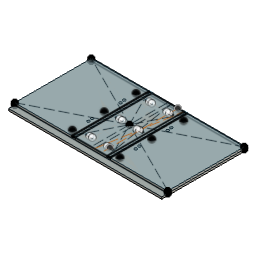
Table Saw Sled v13 (Autodesk Fusion 360 design; units mm, degrees)
Autodesk Fusion 360 part; units mm, degrees
sketch "Sketch1" plane through (0, 0, 0) normal (0, 0, 1) x (1, 0, 0)
  line L0 (0, 0) -> (914.4, 0)
  line L1 (914.4, 0) -> (914.4, 511.2)
  line L2 (914.4, 511.2) -> (0, 511.2)
  line L3 (0, 511.2) -> (0, 0)
  dimension "d1" = 914.4
  dimension "d2" = 511.2
  constraint horizontal L0
  constraint vertical L1
  constraint horizontal L2
  constraint vertical L3
  constraint coincident L0.start L3.end
  measures "d1" distance of L0.start L0.end
  measures "d2" distance of L0.start L2.end
extrude "Extrude1" add sketch "Sketch1" along normal blind 12 makes body 1
sketch "Sketch2" plane through (0, 0, 12) normal (0, 0, 1) x (-1, 0, 0)
  line L0 (0, -511.2) -> (0, 0)
  line L1 (0, 0) -> (-914.4, 0)
  line L2 (-914.4, 0) -> (-914.4, -511.2)
  line L3 (-914.4, -511.2) -> (0, -511.2)
  line L4 (0, 0) -> (-914.4, -511.2) construction
  line L5 (0, -511.2) -> (-914.4, 0) construction
  line L6 (-457.2, -511.2) -> (-457.2, 0) construction
  line L7 (-599.2812, -30.175) -> (-315.1187, -30.175) construction
  line L8 (-315.1187, -30.175) -> (-315.1187, -481.025) construction
  line L9 (-315.1187, -481.025) -> (-599.2812, -481.025) construction
  line L10 (-599.2812, -481.025) -> (-599.2812, -30.175) construction
  line L11 (-599.2812, -30.175) -> (-315.1187, -481.025) construction
  line L12 (-315.1187, -30.175) -> (-599.2812, -481.025) construction
  line L13 (-310.3562, -442.925) -> (-319.8812, -442.925)
  line L14 (-319.8812, -442.925) -> (-319.8812, -449.275)
  line L15 (-319.8812, -449.275) -> (-310.3562, -449.275)
  line L16 (-310.3562, -449.275) -> (-310.3562, -442.925)
  line L17 (-310.3562, -442.925) -> (-319.8812, -449.275) construction
  line L18 (-319.8812, -442.925) -> (-310.3562, -449.275) construction
  line L19 (-604.0438, -442.925) -> (-594.5188, -449.275) construction
  line L20 (-594.5188, -442.925) -> (-604.0438, -449.275) construction
  line L21 (-604.0438, -442.925) -> (-594.5188, -442.925)
  line L22 (-594.5188, -442.925) -> (-594.5188, -449.275)
  line L23 (-604.0438, -449.275) -> (-604.0438, -442.925)
  line L24 (-594.5188, -449.275) -> (-604.0438, -449.275)
  line L25 (-310.3562, -252.425) -> (-319.8812, -252.425)
  line L26 (-319.8812, -252.425) -> (-319.8812, -258.775)
  line L27 (-310.3562, -258.775) -> (-310.3562, -252.425)
  line L28 (-319.8812, -258.775) -> (-310.3562, -258.775)
  line L29 (-310.3562, -252.425) -> (-319.8812, -258.775) construction
  line L30 (-319.8812, -252.425) -> (-310.3562, -258.775) construction
  line L31 (-310.3562, -61.925) -> (-319.8812, -61.925)
  line L32 (-319.8812, -61.925) -> (-319.8812, -68.275)
  line L33 (-310.3562, -68.275) -> (-310.3562, -61.925)
  line L34 (-319.8812, -68.275) -> (-310.3562, -68.275)
  line L35 (-310.3562, -61.925) -> (-319.8812, -68.275) construction
  line L36 (-319.8812, -61.925) -> (-310.3562, -68.275) construction
  line L37 (-604.0438, -252.425) -> (-594.5188, -252.425)
  line L38 (-594.5188, -252.425) -> (-594.5188, -258.775)
  line L39 (-594.5188, -258.775) -> (-604.0438, -258.775)
  line L40 (-604.0438, -258.775) -> (-604.0438, -252.425)
  line L41 (-604.0438, -252.425) -> (-594.5188, -258.775) construction
  line L42 (-594.5188, -252.425) -> (-604.0438, -258.775) construction
  line L43 (-604.0438, -61.925) -> (-594.5188, -61.925)
  line L44 (-594.5188, -61.925) -> (-594.5188, -68.275)
  line L45 (-594.5188, -68.275) -> (-604.0438, -68.275)
  line L46 (-604.0438, -68.275) -> (-604.0438, -61.925)
  line L47 (-604.0438, -61.925) -> (-594.5188, -68.275) construction
  line L48 (-594.5188, -61.925) -> (-604.0438, -68.275) construction
  circle A0 centre (-316.7062, -350.85) radius 7.9375
  circle A1 centre (-316.7062, -160.35) radius 7.9375
  circle A2 centre (-313.5312, -185.75) radius 7.9375
  circle A3 centre (-313.5312, -376.25) radius 7.9375
  circle A4 centre (-597.6938, -374.25) radius 7.9375
  circle A5 centre (-600.8688, -348.85) radius 7.9375
  circle A6 centre (-597.6938, -183.75) radius 7.9375
  circle A7 centre (-600.8688, -158.35) radius 7.9375
  line L49 (-914.4, -255.6) -> (0, -255.6) construction
  line L50 (-31.75, -192.1) -> (-63.5, -192.1)
  line L51 (-63.5, -192.1) -> (-63.5, -319.1)
  line L52 (-63.5, -319.1) -> (-31.75, -319.1)
  line L53 (-31.75, -319.1) -> (-31.75, -192.1)
  line L54 (-31.75, -192.1) -> (-63.5, -319.1) construction
  line L55 (-63.5, -192.1) -> (-31.75, -319.1) construction
  line L56 (-882.65, -319.1) -> (-882.65, -192.1)
  line L57 (-882.65, -192.1) -> (-850.9, -192.1)
  line L58 (-850.9, -319.1) -> (-882.65, -319.1)
  line L59 (-850.9, -192.1) -> (-850.9, -319.1)
  line L60 (-850.9, -192.1) -> (-882.65, -319.1) construction
  line L61 (-882.65, -192.1) -> (-850.9, -319.1) construction
  point P0 (-457.2, -255.6)
  point P1 (-315.1187, -446.1)
  point P2 (-315.1187, -255.6)
  point P3 (-315.1187, -65.1)
  point P4 (-47.625, -255.6)
  point P5 (-866.775, -255.6)
  dimension "d5" = 284.1625
  dimension "d6" = 450.85
  dimension "d7" = 9.525
  dimension "d8" = 6.35
  dimension "d9" = 34.925
  dimension "d12" = 0
  dimension "d13" = 381
  dimension "d16" = 0
  dimension "d17" = 381
  dimension "d18" = 15.875
  dimension "d19" = 95.25
  dimension "d20" = 1.5875
  dimension "d21" = 15.875
  dimension "d22" = 95.25
  dimension "d23" = 1.5875
  dimension "d24" = 15.875
  dimension "d25" = 15.875
  dimension "d26" = 1.5875
  dimension "d27" = 1.5875
  dimension "d28" = 25.4
  dimension "d29" = 25.4
  dimension "d30" = 15.875
  dimension "d31" = 15.875
  dimension "d32" = 25.4
  dimension "d33" = 3.175
  dimension "d34" = 1.5875
  dimension "d35" = 15.875
  dimension "d36" = 15.875
  dimension "d37" = 25.4
  dimension "d38" = 3.175
  dimension "d39" = 1.5875
  dimension "d94" = 31.75
  dimension "d95" = 127
  dimension "d96" = 31.75
  constraint coincident L0.end L1.start
  constraint coincident L2.end L3.start
  constraint coincident L0.start L3.end
  constraint coincident L1.end L2.start
  constraint midpoint L3 L6.start
  constraint midpoint L1 L6.end
  constraint horizontal L7
  constraint perpendicular L7 L8
  constraint parallel L7 L9
  constraint parallel L8 L10
  constraint coincident L11 P0
  constraint coincident L12 P0
  constraint midpoint L5 P0
  constraint horizontal L13
  constraint perpendicular L13 L14
  constraint parallel L13 L15
  constraint parallel L14 L16
  constraint coincident L17 P1
  constraint coincident L18 P1
  constraint coincident L8 P1
  constraint symmetric L6 L13.start L19.start
  constraint symmetric L6 L13.end L20.start
  constraint symmetric L6 L14.end L19.end
  constraint symmetric L6 L15.end L20.end
  constraint midpoint L2 L49.start
  constraint midpoint L0 L49.end
  constraint horizontal L50
  constraint perpendicular L50 L51
  constraint parallel L50 L52
  constraint parallel L51 L53
  constraint coincident L54 P4
  constraint coincident L55 P4
  constraint coincident L49 P4
  constraint symmetric L6 L50.start L56.end
  constraint symmetric L6 L50.end L57.end
  constraint symmetric L6 L51.end L58.start
  constraint symmetric L6 L52.end L56.start
  constraint symmetric L6 P4 P5
  measures "d5" distance of L8.end L9.end
  measures "d6" distance of L7.end L8.end
  measures "d7" distance of L14.end L15.end
  measures "d8" distance of L13.end L14.end
  measures "d9" distance of L8.end P1
  measures "d18" diameter of A0
  measures "d19" vertical distance of P1 A0.centre
  measures "d20" distance of L8 A0.centre
  measures "d21" diameter of A1
  measures "d22" vertical distance of P3 A1.centre
  measures "d23" distance of L8 A1.centre
  measures "d24" diameter of A2
  measures "d25" diameter of A3
  measures "d26" distance of L8 A3.centre
  measures "d27" distance of L8 A2.centre
  measures "d28" vertical distance of A0.centre A3.centre
  measures "d29" vertical distance of A1.centre A2.centre
  measures "d30" diameter of A5
  measures "d31" diameter of A4
  measures "d32" vertical distance of A5.centre A4.centre
  measures "d33" horizontal distance of A5.centre A4.centre
  measures "d34" distance of L10 A4.centre
  measures "d35" diameter of A7
  measures "d36" diameter of A6
  measures "d37" vertical distance of A7.centre A6.centre
  measures "d38" horizontal distance of A7.centre A6.centre
  measures "d39" distance of L10 A6.centre
  measures "d94" distance of L51.end L52.end
  measures "d95" distance of L50.end L51.end
  measures "d96" distance of L0 L52.end
extrude "Extrude2" cut sketch "Sketch2" along normal through all and the other way through all contours L13 L14 L15 L16 | L21 L22 L23 L24 | L25 L26 L27 L28 | L31 L32 L33 L34 | L37 L38 L39 L40 | L43 L44 L45 L46 | A0 | A1 | A2 | A3 | A4 | A5 | A6 | A7 bodies 1
fillet "Fillet1" radius 3.175 24 edges at (310.3562, 449.275, 6) (310.3562, 258.775, 6) (594.5188, 258.775, 6) (594.5188, 449.275, 6) (310.3562, 68.275, 6) (594.5188, 68.275, 6) (319.8812, 61.925, 6) (604.0438, 61.925, 6) (604.0438, 252.425, 6) (604.0438, 442.925, 6) (319.8812, 442.925, 6) (319.8812, 252.425, 6) (604.0438, 258.775, 6) (319.8812, 258.775, 6) (319.8812, 68.275, 6) (319.8812, 449.275, 6) (604.0438, 449.275, 6) (604.0438, 68.275, 6) (310.3562, 252.425, 6) (310.3562, 442.925, 6) (594.5188, 442.925, 6) (594.5188, 252.425, 6) (594.5188, 61.925, 6) (310.3562, 61.925, 6) on bodies 1
copy_body "Body->Comp1" bodies 1 removing the originals makes body 2 in component "Component"
sketch "Sketch1 (2)" plane through (0, 0, 12) normal (0, 0, 1) x (-1, 0, 0) in component "Component'"
  circle A0 centre (-316.7062, -160.35) radius 7.9375
  arc A1 (-600.8688, -252.425) -> (-600.8688, -258.775) centre (-600.8688, -255.6) ccw
  line L0 (-600.8688, -252.425) -> (-597.6938, -252.425)
  arc A2 (-597.6938, -258.775) -> (-597.6938, -252.425) centre (-597.6938, -255.6) ccw
  line L1 (-597.6938, -258.775) -> (-600.8688, -258.775)
  line L2 (-313.5312, -449.275) -> (-316.7062, -449.275)
  arc A3 (-316.7062, -442.925) -> (-316.7062, -449.275) centre (-316.7062, -446.1) ccw
  line L3 (-316.7062, -442.925) -> (-313.5312, -442.925)
  arc A4 (-313.5312, -449.275) -> (-313.5312, -442.925) centre (-313.5312, -446.1) ccw
  circle A5 centre (-597.6938, -374.25) radius 7.9375
  circle A6 centre (-313.5312, -376.25) radius 7.9375
  circle A7 centre (-597.6938, -183.75) radius 7.9375
  arc A8 (-600.8688, -61.925) -> (-600.8688, -68.275) centre (-600.8688, -65.1) ccw
  line L4 (-600.8688, -61.925) -> (-597.6938, -61.925)
  arc A9 (-597.6938, -68.275) -> (-597.6938, -61.925) centre (-597.6938, -65.1) ccw
  line L5 (-597.6938, -68.275) -> (-600.8688, -68.275)
  circle A10 centre (-313.5312, -185.75) radius 7.9375
  arc A11 (-316.7062, -252.425) -> (-316.7062, -258.775) centre (-316.7062, -255.6) ccw
  line L6 (-316.7062, -252.425) -> (-313.5312, -252.425)
  arc A12 (-313.5312, -258.775) -> (-313.5312, -252.425) centre (-313.5312, -255.6) ccw
  line L7 (-313.5312, -258.775) -> (-316.7062, -258.775)
  line L8 (-597.6938, -449.275) -> (-600.8688, -449.275)
  arc A13 (-600.8688, -442.925) -> (-600.8688, -449.275) centre (-600.8688, -446.1) ccw
  line L9 (-600.8688, -442.925) -> (-597.6938, -442.925)
  arc A14 (-597.6938, -449.275) -> (-597.6938, -442.925) centre (-597.6938, -446.1) ccw
  circle A15 centre (-600.8688, -348.85) radius 7.9375
  circle A16 centre (-316.7062, -350.85) radius 7.9375
  circle A17 centre (-600.8688, -158.35) radius 7.9375
  arc A18 (-316.7062, -61.925) -> (-316.7062, -68.275) centre (-316.7062, -65.1) ccw
  line L10 (-316.7062, -61.925) -> (-313.5312, -61.925)
  arc A19 (-313.5312, -68.275) -> (-313.5312, -61.925) centre (-313.5312, -65.1) ccw
  line L11 (-313.5312, -68.275) -> (-316.7062, -68.275)
  line L12 (0, -511.2) -> (0, 0)
  line L13 (0, 0) -> (-914.4, 0)
  line L14 (-914.4, 0) -> (-914.4, -511.2)
  line L15 (-914.4, -511.2) -> (0, -511.2)
  line L16 (0, 0) -> (-914.4, 0)
  line L17 (-914.4, 0) -> (-914.4, -36)
  line L18 (-914.4, -36) -> (0, -36)
  line L19 (0, -36) -> (0, 0)
  dimension "d44" = 914.4
  dimension "d45" = 36
  constraint horizontal L16
  constraint vertical L17
  constraint horizontal L18
  constraint vertical L19
  constraint coincident L12.end L13.start
  measures "d44" distance of L12.end L13.end
  measures "d45" distance of L12.end L18.end
extrude "Extrude1'" add sketch "Sketch1 (2)" along normal blind 101.6 separate body contours L12 L13 L14 L16 L17 L18 L19 makes body 3 in component "Component'"
sketch "Sketch2 (2)" plane through (0, 0, 113.6) normal (0, 0, 1) x (-1, 0, 0) in component "Component'"
  line L0 (0, -36) -> (0, 0)
  line L1 (0, 0) -> (-914.4, 0)
  line L2 (-914.4, 0) -> (-914.4, -36)
  line L3 (-914.4, -36) -> (0, -36)
  line L4 (0, 0) -> (-914.4, -36) construction
  line L5 (-914.4, 0) -> (0, -36) construction
  line L6 (0, -18) -> (-914.4, -18)
  constraint coincident L0.end L1.start
  constraint coincident L2.end L3.start
  constraint coincident L1.end L2.start
  constraint coincident L0.start L3.end
  constraint midpoint L0 L6.start
  constraint midpoint L2 L6.end
extrude "Extrude2'" cut sketch "Sketch2 (2)" against normal blind 9.525 contours L0 L1 L2 L6 bodies 3 in component "Component'"
sketch "Sketch3" plane through (0, 0, 12) normal (0, 0, 1) x (-1, 0, 0) in component "Component'"
  circle A0 centre (-316.7062, -160.35) radius 7.9375
  arc A1 (-600.8688, -252.425) -> (-600.8688, -258.775) centre (-600.8688, -255.6) ccw
  line L0 (-600.8688, -252.425) -> (-597.6938, -252.425)
  arc A2 (-597.6938, -258.775) -> (-597.6938, -252.425) centre (-597.6938, -255.6) ccw
  line L1 (-597.6938, -258.775) -> (-600.8688, -258.775)
  line L2 (-313.5312, -449.275) -> (-316.7062, -449.275)
  arc A3 (-316.7062, -442.925) -> (-316.7062, -449.275) centre (-316.7062, -446.1) ccw
  line L3 (-316.7062, -442.925) -> (-313.5312, -442.925)
  arc A4 (-313.5312, -449.275) -> (-313.5312, -442.925) centre (-313.5312, -446.1) ccw
  circle A5 centre (-597.6938, -374.25) radius 7.9375
  circle A6 centre (-313.5312, -376.25) radius 7.9375
  circle A7 centre (-597.6938, -183.75) radius 7.9375
  arc A8 (-600.8688, -61.925) -> (-600.8688, -68.275) centre (-600.8688, -65.1) ccw
  line L4 (-600.8688, -61.925) -> (-597.6938, -61.925)
  arc A9 (-597.6938, -68.275) -> (-597.6938, -61.925) centre (-597.6938, -65.1) ccw
  line L5 (-597.6938, -68.275) -> (-600.8688, -68.275)
  circle A10 centre (-313.5312, -185.75) radius 7.9375
  arc A11 (-316.7062, -252.425) -> (-316.7062, -258.775) centre (-316.7062, -255.6) ccw
  line L6 (-316.7062, -252.425) -> (-313.5312, -252.425)
  arc A12 (-313.5312, -258.775) -> (-313.5312, -252.425) centre (-313.5312, -255.6) ccw
  line L7 (-313.5312, -258.775) -> (-316.7062, -258.775)
  line L8 (-597.6938, -449.275) -> (-600.8688, -449.275)
  arc A13 (-600.8688, -442.925) -> (-600.8688, -449.275) centre (-600.8688, -446.1) ccw
  line L9 (-600.8688, -442.925) -> (-597.6938, -442.925)
  arc A14 (-597.6938, -449.275) -> (-597.6938, -442.925) centre (-597.6938, -446.1) ccw
  circle A15 centre (-600.8688, -348.85) radius 7.9375
  circle A16 centre (-316.7062, -350.85) radius 7.9375
  circle A17 centre (-600.8688, -158.35) radius 7.9375
  arc A18 (-316.7062, -61.925) -> (-316.7062, -68.275) centre (-316.7062, -65.1) ccw
  line L10 (-316.7062, -61.925) -> (-313.5312, -61.925)
  arc A19 (-313.5312, -68.275) -> (-313.5312, -61.925) centre (-313.5312, -65.1) ccw
  line L11 (-313.5312, -68.275) -> (-316.7062, -68.275)
  line L12 (0, -511.2) -> (0, 0)
  line L13 (0, 0) -> (-914.4, 0)
  line L14 (-914.4, 0) -> (-914.4, -511.2)
  line L15 (-914.4, -511.2) -> (0, -511.2)
  line L16 (0, -511.2) -> (-914.4, -511.2)
  line L17 (-914.4, -511.2) -> (-914.4, -493.2)
  line L18 (-914.4, -493.2) -> (0, -493.2)
  line L19 (0, -493.2) -> (0, -511.2)
  dimension "d50" = 914.4
  dimension "d51" = 18
  constraint horizontal L16
  constraint vertical L17
  constraint horizontal L18
  constraint vertical L19
  constraint coincident L12.start L15.end
  measures "d50" distance of L12.start L14.end
  measures "d51" distance of L12.start L18.end
extrude "Extrude3" add sketch "Sketch3" along normal blind 101.6 separate body contours L12 L14 L15 L16 L17 L18 L19 makes body 4 in component "Component'"
sketch "Sketch4" plane through (0, 511.2, 0) normal (0, 1, 0) x (-1, 0, 0) in component "Component'"
  line L0 (-914.4, 12) -> (0, 12)
  line L1 (0, 12) -> (0, 113.6)
  line L2 (0, 113.6) -> (-914.4, 113.6)
  line L3 (-914.4, 113.6) -> (-914.4, 12)
  line L4 (-406.4, 12) -> (-508, 12)
  line L5 (-508, 12) -> (-508, 113.6)
  line L6 (-508, 113.6) -> (-406.4, 113.6)
  line L7 (-406.4, 113.6) -> (-406.4, 12)
  line L8 (-406.4, 12) -> (-508, 113.6) construction
  line L9 (-508, 12) -> (-406.4, 113.6) construction
  line L10 (-508, 113.6) -> (-558.8, 62.8)
  line L11 (-508, 113.6) -> (-436.158, 113.6) construction
  line L12 (-558.8, 62.8) -> (-914.4, 62.8)
  line L13 (-406.4, 113.6) -> (-355.6, 62.8)
  line L14 (-355.6, 62.8) -> (0, 62.8)
  point P0 (-457.2, 62.8)
  dimension "d54" = 101.6
  dimension "d55" = 135
  constraint horizontal L4
  constraint perpendicular L4 L5
  constraint parallel L4 L6
  constraint parallel L5 L7
  constraint coincident L8 P0
  constraint coincident L9 P0
  constraint horizontal L11
  constraint midpoint L3 L12.end
  constraint perpendicular L3 L12
  constraint perpendicular L9 L13
  constraint midpoint L1 L14.end
  constraint perpendicular L1 L14
  measures "d54" distance of L5.end L6.end
  measures "d55" angle of L10 L11
extrude "Extrude4" cut sketch "Sketch4" along normal through all and the other way up to surface (18 mm away) contours L2 L3 L10 L12 | L1 L2 L13 L14 bodies 4 in component "Component'"
sketch "Sketch2 (3)" plane through (0, 0, 12) normal (0, 0, 1) x (-1, 0, 0) in component "Component''"
  circle A0 centre (-316.7062, -160.35) radius 7.9375
  arc A1 (-600.8688, -252.425) -> (-600.8688, -258.775) centre (-600.8688, -255.6) ccw
  line L0 (-600.8688, -252.425) -> (-597.6938, -252.425)
  arc A2 (-597.6938, -258.775) -> (-597.6938, -252.425) centre (-597.6938, -255.6) ccw
  line L1 (-597.6938, -258.775) -> (-600.8688, -258.775)
  line L2 (-313.5312, -449.275) -> (-316.7062, -449.275)
  arc A3 (-316.7062, -442.925) -> (-316.7062, -449.275) centre (-316.7062, -446.1) ccw
  line L3 (-316.7062, -442.925) -> (-313.5312, -442.925)
  arc A4 (-313.5312, -449.275) -> (-313.5312, -442.925) centre (-313.5312, -446.1) ccw
  circle A5 centre (-597.6938, -374.25) radius 7.9375
  circle A6 centre (-313.5312, -376.25) radius 7.9375
  circle A7 centre (-597.6938, -183.75) radius 7.9375
  arc A8 (-600.8688, -61.925) -> (-600.8688, -68.275) centre (-600.8688, -65.1) ccw
  line L4 (-600.8688, -61.925) -> (-597.6938, -61.925)
  arc A9 (-597.6938, -68.275) -> (-597.6938, -61.925) centre (-597.6938, -65.1) ccw
  line L5 (-597.6938, -68.275) -> (-600.8688, -68.275)
  circle A10 centre (-313.5312, -185.75) radius 7.9375
  arc A11 (-316.7062, -252.425) -> (-316.7062, -258.775) centre (-316.7062, -255.6) ccw
  line L6 (-316.7062, -252.425) -> (-313.5312, -252.425)
  arc A12 (-313.5312, -258.775) -> (-313.5312, -252.425) centre (-313.5312, -255.6) ccw
  line L7 (-313.5312, -258.775) -> (-316.7062, -258.775)
  line L8 (-597.6938, -449.275) -> (-600.8688, -449.275)
  arc A13 (-600.8688, -442.925) -> (-600.8688, -449.275) centre (-600.8688, -446.1) ccw
  line L9 (-600.8688, -442.925) -> (-597.6938, -442.925)
  arc A14 (-597.6938, -449.275) -> (-597.6938, -442.925) centre (-597.6938, -446.1) ccw
  circle A15 centre (-600.8688, -348.85) radius 7.9375
  circle A16 centre (-316.7062, -350.85) radius 7.9375
  circle A17 centre (-600.8688, -158.35) radius 7.9375
  arc A18 (-316.7062, -61.925) -> (-316.7062, -68.275) centre (-316.7062, -65.1) ccw
  line L10 (-316.7062, -61.925) -> (-313.5312, -61.925)
  arc A19 (-313.5312, -68.275) -> (-313.5312, -61.925) centre (-313.5312, -65.1) ccw
  line L11 (-313.5312, -68.275) -> (-316.7062, -68.275)
  line L12 (0, -511.2) -> (0, 0)
  line L13 (0, 0) -> (-914.4, 0)
  line L14 (-914.4, 0) -> (-914.4, -511.2)
  line L15 (-914.4, -511.2) -> (0, -511.2)
  line L16 (0, -493.2) -> (-914.4, -493.2)
  line L17 (0, -36) -> (-914.4, -36)
  dimension "d60" = 36
  dimension "d61" = 18
  constraint coincident L12 L16.start
  constraint coincident L14 L16.end
  constraint perpendicular L14 L16
  constraint coincident L12 L17.start
  constraint coincident L14 L17.end
  constraint perpendicular L14 L17
  measures "d60" distance of L13 L17
  measures "d61" distance of L15 L16
extrude "Extrude1''" add sketch "Sketch2 (3)" along normal blind 12.7 separate body contours L12 L14 L16 L17 makes body 5 in component "Component''"
sketch "Sketch3 (2)" plane through (0, 0, 24.7) normal (0, 0, 1) x (-1, 0, 0) in component "Component''"
  circle A0 centre (-597.6938, -183.75) radius 7.9375
  arc A1 (-600.8688, -252.425) -> (-600.8688, -258.775) centre (-600.8688, -255.6) ccw
  line L0 (-600.8688, -252.425) -> (-597.6938, -252.425)
  arc A2 (-597.6938, -258.775) -> (-597.6938, -252.425) centre (-597.6938, -255.6) ccw
  line L1 (-597.6938, -258.775) -> (-600.8688, -258.775)
  arc A3 (-600.8688, -442.925) -> (-600.8688, -449.275) centre (-600.8688, -446.1) ccw
  line L2 (-600.8688, -442.925) -> (-597.6938, -442.925)
  arc A4 (-597.6938, -449.275) -> (-597.6938, -442.925) centre (-597.6938, -446.1) ccw
  line L3 (-597.6938, -449.275) -> (-600.8688, -449.275)
  circle A5 centre (-316.7062, -160.35) radius 7.9375
  circle A6 centre (-600.8688, -158.35) radius 7.9375
  arc A7 (-316.7062, -61.925) -> (-316.7062, -68.275) centre (-316.7062, -65.1) ccw
  line L4 (-316.7062, -61.925) -> (-313.5312, -61.925)
  arc A8 (-313.5312, -68.275) -> (-313.5312, -61.925) centre (-313.5312, -65.1) ccw
  line L5 (-313.5312, -68.275) -> (-316.7062, -68.275)
  arc A9 (-316.7062, -252.425) -> (-316.7062, -258.775) centre (-316.7062, -255.6) ccw
  line L6 (-316.7062, -252.425) -> (-313.5312, -252.425)
  arc A10 (-313.5312, -258.775) -> (-313.5312, -252.425) centre (-313.5312, -255.6) ccw
  line L7 (-313.5312, -258.775) -> (-316.7062, -258.775)
  circle A11 centre (-313.5312, -185.75) radius 7.9375
  arc A12 (-600.8688, -61.925) -> (-600.8688, -68.275) centre (-600.8688, -65.1) ccw
  line L8 (-600.8688, -61.925) -> (-597.6938, -61.925)
  arc A13 (-597.6938, -68.275) -> (-597.6938, -61.925) centre (-597.6938, -65.1) ccw
  line L9 (-597.6938, -68.275) -> (-600.8688, -68.275)
  circle A14 centre (-313.5312, -376.25) radius 7.9375
  circle A15 centre (-316.7062, -350.85) radius 7.9375
  arc A16 (-316.7062, -442.925) -> (-316.7062, -449.275) centre (-316.7062, -446.1) ccw
  line L10 (-316.7062, -442.925) -> (-313.5312, -442.925)
  arc A17 (-313.5312, -449.275) -> (-313.5312, -442.925) centre (-313.5312, -446.1) ccw
  line L11 (-313.5312, -449.275) -> (-316.7062, -449.275)
  circle A18 centre (-600.8688, -348.85) radius 7.9375
  circle A19 centre (-597.6938, -374.25) radius 7.9375
  line L12 (0, -493.2) -> (0, -36)
  line L13 (0, -36) -> (-914.4, -36)
  line L14 (-914.4, -36) -> (-914.4, -493.2)
  line L15 (-914.4, -493.2) -> (0, -493.2)
  arc A20 (-597.6938, -452.45) -> (-597.6938, -439.75) centre (-597.6938, -446.1) ccw
  line L16 (-600.8688, -439.75) -> (-597.6938, -439.75)
  arc A21 (-600.8688, -439.75) -> (-600.8688, -452.45) centre (-600.8688, -446.1) ccw
  line L17 (-597.6938, -452.45) -> (-600.8688, -452.45)
  arc A22 (-313.5312, -261.95) -> (-313.5312, -249.25) centre (-313.5312, -255.6) ccw
  line L18 (-316.7062, -249.25) -> (-313.5312, -249.25)
  arc A23 (-316.7062, -249.25) -> (-316.7062, -261.95) centre (-316.7062, -255.6) ccw
  line L19 (-313.5312, -261.95) -> (-316.7062, -261.95)
  arc A24 (-597.6938, -71.45) -> (-597.6938, -58.75) centre (-597.6938, -65.1) ccw
  line L20 (-600.8688, -58.75) -> (-597.6938, -58.75)
  arc A25 (-600.8688, -58.75) -> (-600.8688, -71.45) centre (-600.8688, -65.1) ccw
  line L21 (-597.6938, -71.45) -> (-600.8688, -71.45)
  arc A26 (-313.5312, -71.45) -> (-313.5312, -58.75) centre (-313.5312, -65.1) ccw
  line L22 (-316.7062, -58.75) -> (-313.5312, -58.75)
  arc A27 (-316.7062, -58.75) -> (-316.7062, -71.45) centre (-316.7062, -65.1) ccw
  line L23 (-313.5312, -71.45) -> (-316.7062, -71.45)
  arc A28 (-313.5312, -452.45) -> (-313.5312, -439.75) centre (-313.5312, -446.1) ccw
  line L24 (-316.7062, -439.75) -> (-313.5312, -439.75)
  arc A29 (-316.7062, -439.75) -> (-316.7062, -452.45) centre (-316.7062, -446.1) ccw
  line L25 (-313.5312, -452.45) -> (-316.7062, -452.45)
  arc A30 (-597.6938, -261.95) -> (-597.6938, -249.25) centre (-597.6938, -255.6) ccw
  line L26 (-600.8688, -249.25) -> (-597.6938, -249.25)
  arc A31 (-600.8688, -249.25) -> (-600.8688, -261.95) centre (-600.8688, -255.6) ccw
  line L27 (-597.6938, -261.95) -> (-600.8688, -261.95)
  dimension "d64" = -3.175
  measures "d64" distance of A4
extrude "Extrude2''" cut sketch "Sketch3 (2)" along normal blind -4.7625 and the other way blind 0 contours A20 L16 A21 L17 | A22 L18 A23 L19 | A24 L20 A25 L21 | A26 L22 A27 L23 | A28 L24 A29 L25 | A30 L26 A31 L27 bodies 5 in component "Component''"
sketch "Sketch4 (2)" plane through (0, 0, 24.7) normal (0, 0, 1) x (-1, 0, 0) in component "Component''"
  line L0 (-597.6938, -452.45) -> (-600.8688, -452.45)
  arc A0 (-600.8688, -439.75) -> (-600.8688, -452.45) centre (-600.8688, -446.1) ccw
  line L1 (-600.8688, -439.75) -> (-597.6938, -439.75)
  arc A1 (-597.6938, -452.45) -> (-597.6938, -439.75) centre (-597.6938, -446.1) ccw
  line L2 (-313.5312, -71.45) -> (-316.7062, -71.45)
  arc A2 (-316.7062, -58.75) -> (-316.7062, -71.45) centre (-316.7062, -65.1) ccw
  line L3 (-316.7062, -58.75) -> (-313.5312, -58.75)
  arc A3 (-313.5312, -71.45) -> (-313.5312, -58.75) centre (-313.5312, -65.1) ccw
  line L4 (-313.5312, -452.45) -> (-316.7062, -452.45)
  arc A4 (-316.7062, -439.75) -> (-316.7062, -452.45) centre (-316.7062, -446.1) ccw
  line L5 (-316.7062, -439.75) -> (-313.5312, -439.75)
  arc A5 (-313.5312, -452.45) -> (-313.5312, -439.75) centre (-313.5312, -446.1) ccw
  line L6 (-597.6938, -261.95) -> (-600.8688, -261.95)
  arc A6 (-600.8688, -249.25) -> (-600.8688, -261.95) centre (-600.8688, -255.6) ccw
  line L7 (-600.8688, -249.25) -> (-597.6938, -249.25)
  arc A7 (-597.6938, -261.95) -> (-597.6938, -249.25) centre (-597.6938, -255.6) ccw
  line L8 (-597.6938, -71.45) -> (-600.8688, -71.45)
  arc A8 (-600.8688, -58.75) -> (-600.8687, -71.45) centre (-600.8688, -65.1) ccw
  line L9 (-600.8688, -58.75) -> (-597.6938, -58.75)
  arc A9 (-597.6938, -71.45) -> (-597.6938, -58.75) centre (-597.6938, -65.1) ccw
  line L10 (-313.5312, -261.95) -> (-316.7062, -261.95)
  arc A10 (-316.7062, -249.25) -> (-316.7062, -261.95) centre (-316.7062, -255.6) ccw
  line L11 (-316.7062, -249.25) -> (-313.5312, -249.25)
  arc A11 (-313.5312, -261.95) -> (-313.5312, -249.25) centre (-313.5312, -255.6) ccw
  circle A12 centre (-597.6938, -183.75) radius 7.9375
  circle A13 centre (-316.7062, -160.35) radius 7.9375
  circle A14 centre (-600.8688, -158.35) radius 7.9375
  circle A15 centre (-313.5312, -185.75) radius 7.9375
  circle A16 centre (-313.5312, -376.25) radius 7.9375
  circle A17 centre (-316.7062, -350.85) radius 7.9375
  circle A18 centre (-600.8688, -348.85) radius 7.9375
  circle A19 centre (-597.6938, -374.25) radius 7.9375
  line L12 (0, -493.2) -> (0, -36)
  line L13 (0, -36) -> (-914.4, -36)
  line L14 (-914.4, -36) -> (-914.4, -493.2)
  line L15 (-914.4, -493.2) -> (0, -493.2)
  line L16 (0, -36) -> (-914.4, -493.2) construction
  line L17 (-914.4, -36) -> (0, -493.2) construction
  line L18 (-342.9, -493.2) -> (-571.5, -493.2)
  line L19 (-571.5, -493.2) -> (-571.5, -36)
  line L20 (-571.5, -36) -> (-342.9, -36)
  line L21 (-342.9, -36) -> (-342.9, -493.2)
  line L22 (-342.9, -493.2) -> (-571.5, -36) construction
  line L23 (-571.5, -493.2) -> (-342.9, -36) construction
  line L24 (-571.5, -36) -> (-552.45, -36)
  line L25 (-552.45, -36) -> (-552.45, -494.848)
  line L26 (-552.45, -494.848) -> (-571.5, -494.848)
  line L27 (-571.5, -494.848) -> (-571.5, -36)
  line L28 (-342.9, -36) -> (-361.95, -36)
  line L29 (-361.95, -36) -> (-361.95, -495.1951)
  line L30 (-361.95, -495.1951) -> (-342.9, -495.1951)
  line L31 (-342.9, -495.1951) -> (-342.9, -36)
  line L32 (-457.2, -493.2) -> (-457.2, -36) construction
  line L33 (-476.25, -493.2) -> (-476.25, -36) construction
  line L34 (-476.25, -36) -> (-552.45, -494.848) construction
  line L35 (-476.25, -493.2) -> (-552.45, -36) construction
  line L36 (-517.5749, -493.2) -> (-517.5749, -36) construction
  line L37 (-498.5249, -83.625) -> (-536.6249, -83.625)
  line L38 (-536.6249, -83.625) -> (-536.6249, -89.975)
  line L39 (-536.6249, -89.975) -> (-498.5249, -89.975)
  line L40 (-498.5249, -89.975) -> (-498.5249, -83.625)
  line L41 (-498.5249, -83.625) -> (-536.6249, -89.975) construction
  line L42 (-536.6249, -83.625) -> (-498.5249, -89.975) construction
  line L43 (-377.7751, -89.975) -> (-415.8751, -89.975)
  line L44 (-415.8751, -83.625) -> (-377.7751, -89.975) construction
  line L45 (-377.7751, -83.625) -> (-415.8751, -89.975) construction
  line L46 (-377.7751, -83.625) -> (-377.7751, -89.975)
  line L47 (-415.8751, -83.625) -> (-377.7751, -83.625)
  line L48 (-415.8751, -89.975) -> (-415.8751, -83.625)
  line L49 (-415.8751, -261.425) -> (-377.7751, -261.425)
  line L50 (-377.7751, -261.425) -> (-377.7751, -267.775)
  line L51 (-377.7751, -267.775) -> (-415.8751, -267.775)
  line L52 (-415.8751, -267.775) -> (-415.8751, -261.425)
  line L53 (-415.8751, -261.425) -> (-377.7751, -267.775) construction
  line L54 (-377.7751, -261.425) -> (-415.8751, -267.775) construction
  line L55 (-536.6249, -267.775) -> (-498.5249, -267.775)
  line L56 (-498.5249, -261.425) -> (-536.6249, -267.775) construction
  line L57 (-536.6249, -261.425) -> (-498.5249, -267.775) construction
  line L58 (-415.8751, -439.225) -> (-377.7751, -439.225)
  line L59 (-377.7751, -439.225) -> (-377.7751, -445.575)
  line L60 (-377.7751, -445.575) -> (-415.8751, -445.575)
  line L61 (-415.8751, -445.575) -> (-415.8751, -439.225)
  line L62 (-415.8751, -439.225) -> (-377.7751, -445.575) construction
  line L63 (-377.7751, -439.225) -> (-415.8751, -445.575) construction
  line L64 (-536.6249, -445.575) -> (-498.5249, -445.575)
  line L65 (-498.5249, -439.225) -> (-536.6249, -445.575) construction
  line L66 (-536.6249, -439.225) -> (-498.5249, -445.575) construction
  line L67 (-498.5249, -261.425) -> (-536.6249, -261.425)
  line L68 (-498.5249, -267.775) -> (-498.5249, -261.425)
  line L69 (-536.6249, -261.425) -> (-536.6249, -267.775)
  line L70 (-498.5249, -439.225) -> (-536.6249, -439.225)
  line L71 (-498.5249, -445.575) -> (-498.5249, -439.225)
  line L72 (-536.6249, -439.225) -> (-536.6249, -445.575)
  point P0 (-457.2, -264.6)
  point P1 (-517.5749, -86.8)
  point P2 (-396.8251, -86.8)
  point P3 (-396.8251, -264.6)
  point P4 (-517.5749, -264.6)
  point P5 (-396.8251, -442.4)
  point P6 (-517.5749, -442.4)
  point P7 (-412.7001, -86.8)
  point P8 (-412.7001, -264.6)
  point P9 (-412.7001, -442.4)
  point P10 (-501.6999, -86.8)
  point P11 (-501.6999, -264.6)
  point P12 (-501.6999, -442.4)
  dimension "d69" = 228.6
  dimension "d70" = 457.2
  dimension "d71" = 19.05
  dimension "d72" = 19.05
  dimension "d76" = 19.05
  dimension "d77" = 38.1
  dimension "d78" = 6.35
  dimension "d79" = 50.8
  dimension "d82" = 0
  dimension "d83" = -355.6
  dimension "d107" = 3.175
  constraint coincident L12.end L13.start
  constraint coincident L14.end L15.start
  constraint coincident L13.end L14.start
  constraint coincident L12.start L15.end
  constraint horizontal L18
  constraint perpendicular L18 L19
  constraint parallel L18 L20
  constraint parallel L19 L21
  constraint coincident L22 P0
  constraint coincident L23 P0
  constraint midpoint L16 P0
  constraint horizontal L24
  constraint vertical L25
  constraint horizontal L26
  constraint vertical L27
  constraint horizontal L28
  constraint vertical L29
  constraint horizontal L30
  constraint vertical L31
  constraint midpoint L18 L32.start
  constraint midpoint L20 L32.end
  constraint coincident L18 L33.start
  constraint coincident L20 L33.end
  constraint perpendicular L20 L33
  constraint coincident L15 L36.start
  constraint perpendicular L15 L36
  constraint coincident L20 L36.end
  constraint horizontal L37
  constraint perpendicular L37 L38
  constraint parallel L37 L39
  constraint parallel L38 L40
  constraint coincident L41 P1
  constraint coincident L42 P1
  constraint coincident L36 P1
  constraint symmetric L32 L37.start L44.start
  constraint symmetric L32 L37.end L45.start
  constraint symmetric L32 L38.end L43.start
  constraint symmetric L32 P7 P10
  constraint symmetric L32 P8 P11
  constraint symmetric L32 P9 P12
  measures "d69" distance of L19.end L20.end
  measures "d70" distance of L18.end L19.end
  measures "d71" distance of L19.end L24.end
  measures "d72" distance of L20.end L28.end
  measures "d76" distance of L32 L33
  measures "d77" distance of L38.end L39.end
  measures "d78" distance of L37.end L38.end
  measures "d79" distance of L13 P1
  measures "d107" distance of L48 P7
extrude "Extrude3'" cut sketch "Sketch4 (2)" along normal blind 0 and the other way blind 12.7 contours L13 L15 L18 L20 L21 L28 L29 L31 | L13 L15 L18 L19 L20 L24 L25 L27 | L37 L38 L39 L40 | L43 L46 L47 L48 | L49 L50 L51 L52 | L55 L67 L68 L69 | L58 L59 L60 L61 | L64 L70 L71 L72 bodies 5 makes body 6 at (810.9318, 261.7838, 12) makes body 7 at (470.975, 204.275, 12) in component "Component''"
fillet "Fillet1'" radius 3.175 24 edges at (377.7751, 267.775, 18.35) (377.7751, 445.575, 18.35) (377.7751, 89.975, 18.35) (498.5249, 89.975, 18.35) (498.5249, 267.775, 18.35) (498.5249, 445.575, 18.35) (415.8751, 439.225, 18.35) (536.6249, 439.225, 18.35) (536.6249, 261.425, 18.35) (415.8751, 261.425, 18.35) (415.8751, 83.625, 18.35) (536.6249, 83.625, 18.35) (415.8751, 267.775, 18.35) (536.6249, 267.775, 18.35) (536.6249, 445.575, 18.35) (415.8751, 445.575, 18.35) (415.8751, 89.975, 18.35) (536.6249, 89.975, 18.35) (498.5249, 261.425, 18.35) (377.7751, 261.425, 18.35) (377.7751, 83.625, 18.35) (498.5249, 83.625, 18.35) (498.5249, 439.225, 18.35) (377.7751, 439.225, 18.35) on bodies 7 in component "Component''"
sketch "Sketch5" plane through (0, 0, 24.7) normal (0, 0, 1) x (-1, 0, 0) in component "Component''"
  line L0 (-361.95, -493.2) -> (-361.95, -36)
  line L1 (-361.95, -36) -> (-552.45, -36)
  line L2 (-552.45, -36) -> (-552.45, -493.2)
  line L3 (-552.45, -493.2) -> (-361.95, -493.2)
  line L4 (-501.6999, -267.775) -> (-533.4499, -267.775)
  arc A0 (-533.4499, -261.425) -> (-533.4499, -267.775) centre (-533.4499, -264.6) ccw
  line L5 (-533.4499, -261.425) -> (-501.6999, -261.425)
  arc A1 (-501.6999, -267.775) -> (-501.6999, -261.425) centre (-501.6999, -264.6) ccw
  line L6 (-501.6999, -445.575) -> (-533.4499, -445.575)
  arc A2 (-533.4499, -439.225) -> (-533.4499, -445.575) centre (-533.4499, -442.4) ccw
  line L7 (-533.4499, -439.225) -> (-501.6999, -439.225)
  arc A3 (-501.6999, -445.575) -> (-501.6999, -439.225) centre (-501.6999, -442.4) ccw
  arc A4 (-380.9501, -89.975) -> (-380.9501, -83.625) centre (-380.9501, -86.8) ccw
  line L8 (-380.9501, -89.975) -> (-412.7001, -89.975)
  arc A5 (-412.7001, -83.625) -> (-412.7001, -89.975) centre (-412.7001, -86.8) ccw
  line L9 (-412.7001, -83.625) -> (-380.9501, -83.625)
  arc A6 (-380.9501, -267.775) -> (-380.9501, -261.425) centre (-380.9501, -264.6) ccw
  line L10 (-380.9501, -267.775) -> (-412.7001, -267.775)
  arc A7 (-412.7001, -261.425) -> (-412.7001, -267.775) centre (-412.7001, -264.6) ccw
  line L11 (-412.7001, -261.425) -> (-380.9501, -261.425)
  arc A8 (-380.9501, -445.575) -> (-380.9501, -439.225) centre (-380.9501, -442.4) ccw
  line L12 (-380.9501, -445.575) -> (-412.7001, -445.575)
  arc A9 (-412.7001, -439.225) -> (-412.7001, -445.575) centre (-412.7001, -442.4) ccw
  line L13 (-412.7001, -439.225) -> (-380.9501, -439.225)
  line L14 (-533.4499, -83.625) -> (-501.6999, -83.625)
  arc A10 (-501.6999, -89.975) -> (-501.6999, -83.625) centre (-501.6999, -86.8) ccw
  line L15 (-501.6999, -89.975) -> (-533.4499, -89.975)
  arc A11 (-533.4499, -83.625) -> (-533.4499, -89.975) centre (-533.4499, -86.8) ccw
  line L16 (-412.7001, -436.025) -> (-380.9501, -436.025)
  arc A12 (-380.9501, -448.775) -> (-380.9501, -436.025) centre (-380.9501, -442.4) ccw
  line L17 (-380.9501, -448.775) -> (-412.7001, -448.775)
  arc A13 (-412.7001, -436.025) -> (-412.7001, -448.775) centre (-412.7001, -442.4) ccw
  line L18 (-533.4499, -80.425) -> (-501.6999, -80.425)
  arc A14 (-501.6999, -93.175) -> (-501.6999, -80.425) centre (-501.6999, -86.8) ccw
  line L19 (-501.6999, -93.175) -> (-533.4499, -93.175)
  arc A15 (-533.4499, -80.425) -> (-533.4499, -93.175) centre (-533.4499, -86.8) ccw
  line L20 (-412.7001, -258.225) -> (-380.9501, -258.225)
  arc A16 (-380.9501, -270.975) -> (-380.9501, -258.225) centre (-380.9501, -264.6) ccw
  line L21 (-380.9501, -270.975) -> (-412.7001, -270.975)
  arc A17 (-412.7001, -258.225) -> (-412.7001, -270.975) centre (-412.7001, -264.6) ccw
  line L22 (-533.4499, -258.225) -> (-501.6999, -258.225)
  arc A18 (-501.6999, -270.975) -> (-501.6999, -258.225) centre (-501.6999, -264.6) ccw
  line L23 (-501.6999, -270.975) -> (-533.4499, -270.975)
  arc A19 (-533.4499, -258.225) -> (-533.4499, -270.975) centre (-533.4499, -264.6) ccw
  line L24 (-412.7001, -80.425) -> (-380.9501, -80.425)
  arc A20 (-380.9501, -93.175) -> (-380.9501, -80.425) centre (-380.9501, -86.8) ccw
  line L25 (-380.9501, -93.175) -> (-412.7001, -93.175)
  arc A21 (-412.7001, -80.425) -> (-412.7001, -93.175) centre (-412.7001, -86.8) ccw
  line L26 (-533.4499, -436.025) -> (-501.6999, -436.025)
  arc A22 (-501.6999, -448.775) -> (-501.6999, -436.025) centre (-501.6999, -442.4) ccw
  line L27 (-501.6999, -448.775) -> (-533.4499, -448.775)
  arc A23 (-533.4499, -436.025) -> (-533.4499, -448.775) centre (-533.4499, -442.4) ccw
  dimension "d87" = -3.2
hole "Hole1" at (412.7001, 86.8, 24.7) at (412.7001, 264.6, 24.7) at (501.6999, 264.6, 24.7) at (501.6999, 86.8, 24.7) at (501.6999, 442.4, 24.7) at (412.7001, 442.4, 24.7) direction (0, 0, -1) diameter 9.525 end through all bodies 2 in component "Component"
extrude "Extrude4'" cut sketch "Sketch5" against normal blind 4.7625 contours L16 A12 L17 A13 | L18 A14 L19 A15 | L20 A16 L21 A17 | L22 A18 L23 A19 | L24 A20 L25 A21 | L26 A22 L27 A23 bodies 7 in component "Component''"
component "Component" placed x (1, 0, 0) y (0, 1, 0) z (0, 0, 1) at (0, 0, 0)
component "Component'" placed x (1, 0, 0) y (0, 1, 0) z (0, 0, 1) at (0, 0, 0)
component "Component''" placed x (1, 0, 0) y (0, 1, 0) z (0, 0, 1) at (0, 0, 0)
equation "d5 = 11 3/16\""
equation "d18 = ( 5 / 8 ) * 1 in"
equation "d21 = ( 5 / 8 ) * 1 in"
equation "d24 = ( 5 / 8 ) * 1 in"
equation "d25 = ( 5 / 8 ) * 1 in"
equation "d30 = ( 5 / 8 ) * 1 in"
equation "d31 = ( 5 / 8 ) * 1 in"
equation "d35 = ( 5 / 8 ) * 1 in"
equation "d36 = ( 5 / 8 ) * 1 in"
equation "d65 = ( -3 / 16 ) * 1 in"
equation "d88 = ( -3 / 16 ) * 1 in"
